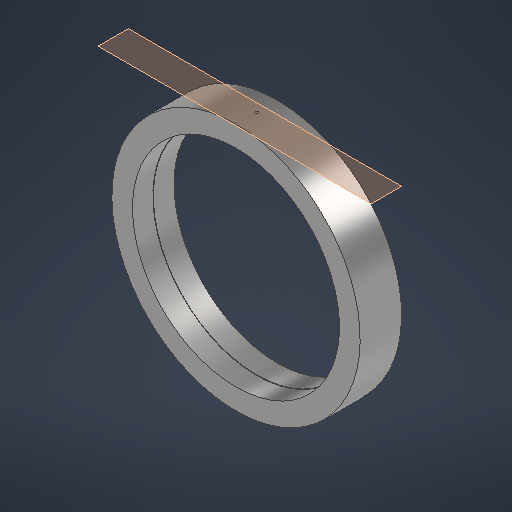
# Autodesk Inventor part: SFD_CuscinettoRadiale180x150x0.20
Saved by Autodesk Inventor 2026.2 (Build 302298010, 298A)
## iProperties
Created: 2026-04-15
Part Number: SFD_CuscinettoRadiale180x150x0.20
Material: Stainless Steel
Document SubType Name: Modeling
Designer: Yan
Density: 8 g/cm^3
Appearance: Semi-Polished
Author: Yan
Autodesk Inventor part; units mm, degrees
ref_plane "YZ Plane" through (0, 0, 0) normal (1, 0, 0) x (0, 1, 0)
ref_plane "XY Plane" through (0, 0, 0) normal (0, 0, 1) x (1, 0, 0)
sketch "Sketch3" plane through (0, 0, 0) normal (1, 0, 0) x (0, 1, 0)
  line L0 (0, 0) -> (0, -30)
  line L1 (0, -30) -> (90, -30)
  line L2 (90, -30) -> (90, 0)
  line L3 (90, 0) -> (0, 0)
  line L4 (75, 0) -> (75, -14.9)
  line L5 (75, -14.9) -> (75.2, -14.9)
  line L6 (75.2, -14.9) -> (75.2, -15.1)
  line L7 (75.2, -15.1) -> (75, -15.1)
  line L8 (75, -15.1) -> (75, -30)
  dimension "d15" = 0.2
  dimension "d16" = 0.2
  dimension "d17" = 180
  dimension "d18" = 150
  dimension "d19" = 14.9
  dimension "d20" = 30
  constraints: 18 end point, 7 perpendicular, 4 point on line, 1 vertical
  measures "d15" distance between parallel lines of L7 L5
  measures "d16" distance of L4.end L5.end
  measures "d17" diameter of L2 L0
  measures "d18" diameter of L4 L0
  measures "d19" distance between parallel lines of L3 L5
  measures "d20" distance of L1.end L2.end
revolve "Revolution2" add sketch "Sketch3" angle 360 about axis through (0, 0, 0) along (0, 0, -1) contours L3 L2 L1 L8 L7 L6 L5 L4
ref_plane "Work Plane2" through (0, 90, 0) normal (0, 1, 0) x (-1, 0, 0)
sketch "Sketch4" plane through (0, 90, 0) normal (0, 1, 0) x (-1, 0, 0)
  line L0 (-75, -14.9) -> (75, -14.9) projected
  point P0 (0, 0)
  point P1 (0.0442, -15)
  dimension "d24" = 15
  measures "d24" vertical distance of point (0, 0) point (0.044, -15)
hole "Hole2" at (-0.0442, 90, -15) direction (0, -1, 0) diameter 2 depth 30 tip angle 118
body "Solid2"
